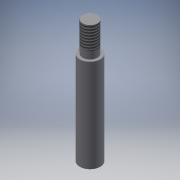
# Autodesk Inventor part: axis5_5
Saved by Autodesk Inventor 2019 (Build 230136000, 136)
## iProperties
Created: 2021-04-07
Part Number: axis5_5
Material: Stainless Steel
Document SubType Name: Modeling
Designer: rtavi
Density: 8 g/cm^3
Appearance: Semi-Polished
Mass: 5.55591 g
Surface Area: 5.80017 cm^2
Volume: 0.694488 cm^3
Author: rtavi
Autodesk Inventor part; units mm, degrees
ref_plane "YZ Plane" through (0, 0, 0) normal (1, 0, 0) x (0, 1, 0)
ref_plane "XZ Plane" through (0, 0, 0) normal (0, 1, 0) x (-1, 0, 0)
ref_plane "XY Plane" through (0, 0, 0) normal (0, 0, 1) x (1, 0, 0)
sketch "Sketch1" plane through (0, 0, 0) normal (0, 1, 0) x (-1, 0, 0)
  circle A0 centre (0, 0) radius 2.75
  dimension "d0" = 5.5
  constraints: 1 centre point, 1 coincident
  measures "d0" diameter of A0
extrude "Extrusion1" add sketch "Sketch1" against normal blind 25
sketch "Sketch2" plane through (0, 0, 0) normal (0, 1, 0) x (-1, 0, 0)
  circle A0 centre (0, 0) radius 2
  dimension "d3" = 4
  constraints: 1 centre point, 1 coincident
  measures "d3" diameter of A0
extrude "Extrusion2" add sketch "Sketch2" along normal blind 8
thread "Thread1" size "M4x0.7" class "6g" standard "ANSI Metric M Profile" length 6
body "Solid1"
